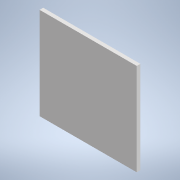
# Autodesk Inventor part: trás
Saved by Autodesk Inventor 2020 (Build 240168000, 168)
## iProperties
Created: 2020-04-24
Part Number: trás
Material: Genérico
Document SubType Name: Modeling
Designer: gi-se
Density: 1 g/cm^3
Appearance: Padrão
Author: gi-se
Autodesk Inventor part; units mm, degrees
ref_plane "YZ Plane" through (0, 0, 0) normal (1, 0, 0) x (0, 1, 0)
ref_plane "XZ Plane" through (0, 0, 0) normal (0, 1, 0) x (-1, 0, 0)
ref_plane "XY Plane" through (0, 0, 0) normal (0, 0, 1) x (1, 0, 0)
sketch "Esboço1" plane through (0, 0, 0) normal (0, 0, 1) x (1, 0, 0)
  line L0 (-50.3718, 0) -> (-50.3718, 1.5) projected
  line L1 (24, 0) -> (24, 1.5) projected
  line L2 (-73.0466, 25.6) -> (-75.024, 25.6) projected
  line L3 (23.9, -47.2) -> (16.1, -47.2) projected
  line L4 (24, 25.6) -> (24, -47.2)
  line L5 (24, -47.2) -> (-56, -47.2)
  line L6 (-56, -47.2) -> (-56, 25.6)
  line L7 (24, 25.6) -> (24, 28.6)
  line L8 (24, 28.6) -> (-56, 28.6)
  line L9 (-56, 28.6) -> (-56, 25.6)
  point P0 (0, 0)
  point P1 (-56, 1.5)
  point P2 (-56, 0)
  dimension "d0" = 80
  constraints: 12 end point, 2 parallel, 1 point on line
  measures "d0" distance of L4.end L5.end
extrude "Extrusão1" add sketch "Esboço1" along normal blind 3
